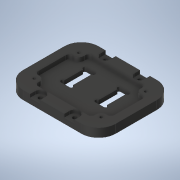
# Autodesk Inventor part: カメラ_メインフレーム1_KCSU5380
Saved by Autodesk Inventor 2020.3 (Build 243373000, 373)
## iProperties
Created: 2018-06-08
Part Number: カメラ_メインフレーム1_KCSU5380
Material: アセタール樹脂、黒
Document SubType Name: Modeling
Designer: taka
Density: 1.425 g/cm^3
Appearance: 滑らか - 黒
Mass: 10.5319 g
Surface Area: 59.4191 cm^2
Volume: 7.39082 cm^3
Category: 頭
Author: taka
Autodesk Inventor part; units mm, degrees
ref_plane "YZ Plane" through (0, 0, 0) normal (1, 0, 0) x (0, 1, 0)
ref_plane "XZ Plane" through (0, 0, 0) normal (0, 1, 0) x (-1, 0, 0)
ref_plane "XY Plane" through (0, 0, 0) normal (0, 0, 1) x (1, 0, 0)
derived "カメラ_メインフレーム1_基礎.ipt"
sketch "スケッチ1" plane through (0, 0, 0) normal (0, 1, 0) x (-1, 0, 0)
  line L0 (0, 0) -> (44, 0)
  line L1 (44, 0) -> (44, -54)
  line L2 (44, -54) -> (0, -54)
  line L3 (0, -54) -> (0, 0)
  line L4 (32.5, -14.5) -> (17.5, -14.5) construction
  line L5 (17.5, -14.5) -> (17.5, -19.5) construction
  line L6 (17.5, -19.5) -> (32.5, -19.5) construction
  line L7 (32.5, -19.5) -> (32.5, -14.5) construction
  line L8 (32.5, -34.5) -> (17.5, -34.5) construction
  line L9 (17.5, -34.5) -> (17.5, -39.5) construction
  line L10 (17.5, -39.5) -> (32.5, -39.5) construction
  line L11 (32.5, -39.5) -> (32.5, -34.5) construction
  line L12 (32.55, -19.55) -> (17.45, -19.55)
  line L13 (17.45, -19.55) -> (17.45, -14.45)
  line L14 (17.45, -14.45) -> (32.55, -14.45)
  line L15 (32.55, -14.45) -> (32.55, -19.55)
  line L16 (17.45, -34.45) -> (32.55, -34.45)
  line L17 (32.55, -34.45) -> (32.55, -39.55)
  line L18 (32.55, -39.55) -> (17.45, -39.55)
  line L19 (17.45, -39.55) -> (17.45, -34.45)
  circle A0 centre (31.5, -19.55) radius 1.05
  circle A1 centre (31.5, -14.45) radius 1.05
  circle A2 centre (18.5, -19.55) radius 1.05
  circle A3 centre (18.5, -14.45) radius 1.05
  circle A4 centre (18.5, -34.45) radius 1.05
  circle A5 centre (18.5, -39.55) radius 1.05
  circle A6 centre (31.5, -34.45) radius 1.05
  circle A7 centre (31.5, -39.55) radius 1.05
  circle A8 centre (35, -7.5) radius 0.8
  circle A9 centre (35, -46.5) radius 0.8
  circle A10 centre (9, -7.5) radius 0.8
  circle A11 centre (9, -46.5) radius 0.8
  circle A12 centre (41, -17) radius 1.15
  circle A13 centre (41, -37) radius 1.15
  line L20 (44, -14.5) -> (0, -14.5) construction
  line L21 (0, -14.5) -> (0, -19.5) construction
  line L22 (0, -19.5) -> (44, -19.5) construction
  line L23 (44, -19.5) -> (44, -14.5)
  circle A14 centre (3, -17) radius 1.15
  circle A15 centre (3, -37) radius 1.15
  line L24 (44, -34.5) -> (0, -34.5) construction
  line L25 (0, -34.5) -> (0, -39.5) construction
  line L26 (0, -39.5) -> (44, -39.5) construction
  line L27 (44, -39.5) -> (44, -34.5)
  line L28 (38, -4.5) -> (6, -4.5) construction
  line L29 (6, -4.5) -> (6, -49.5) construction
  line L30 (6, -49.5) -> (38, -49.5) construction
  line L31 (38, -49.5) -> (38, -4.5) construction
  circle A16 centre (22, -27) radius 7.5 construction
  line L32 (29.5, -13) -> (14.5, -13) construction
  line L33 (14.5, -13) -> (14.5, -53) construction
  line L34 (14.5, -53) -> (29.5, -53) construction
  line L35 (29.5, -53) -> (29.5, -13) construction
  circle A17 centre (22, -27) radius 6.5 construction
  circle A18 centre (26.5, -50) radius 0.9
  circle A19 centre (17.5, -16) radius 0.9
extrude "押し出し1" add sketch "スケッチ1" along normal blind 5 contours L0 L1 L2 L3 | A19 L13 | A18
fillet "フィレット1" radius 10 4 edges at (0, 2.5, -54) (0, 2.5, 0) (-44, 2.5, -54) (-44, 2.5, 0)
sketch "スケッチ4" plane through (-34, 5, 0) normal (0, 1, 0) x (1, 0, 0)
  circle A0 centre (-1, 7.5) radius 3
  circle A1 centre (-1, 46.5) radius 3
  circle A2 centre (25, 46.5) radius 3
  circle A3 centre (25, 7.5) radius 3
  circle A4 centre (-1, 7.5) radius 0.8 projected
  circle A5 centre (-1, 46.5) radius 0.8 projected
  circle A6 centre (25, 46.5) radius 0.8 projected
  circle A7 centre (25, 7.5) radius 0.8 projected
  line L0 (-3.7272, 8.75) -> (-3.7272, 45.25)
  line L1 (27.7272, 8.75) -> (27.7272, 45.25)
  line L2 (0.25, 49.2272) -> (23.75, 49.2272)
  line L3 (0.25, 4.7728) -> (23.75, 4.7728)
  point P0 (34, 0)
  dimension "d16" = 6
  dimension "d17" = 6
  dimension "d18" = 6
  dimension "d19" = 6
  constraints: 8 end point, 8 point on circle, 4 centre point, 4 concentric, 2 parallel, 1 perpendicular, 1 vertical
  measures "d16" diameter of A0
  measures "d17" diameter of A1
  measures "d18" diameter of A2
  measures "d19" diameter of A3
extrude "押し出し4" cut sketch "スケッチ4" against normal blind 2.6 contours A0 L0 A1 L2 A2 L1 A3 L3
sketch "スケッチ5" plane through (-34, 5, 0) normal (0, 1, 0) x (1, 0, 0)
  circle A0 centre (-7, 17) radius 3
  circle A1 centre (-7, 37) radius 3
  circle A2 centre (31, 17) radius 3
  circle A3 centre (31, 37) radius 3
  circle A4 centre (-7, 17) radius 1.15 projected
  circle A5 centre (-7, 37) radius 1.15 projected
  circle A6 centre (31, 37) radius 1.15 projected
  circle A7 centre (31, 17) radius 1.15 projected
  line L0 (-7, 20) -> (-10, 20)
  line L1 (-7, 14) -> (-10, 14)
  line L2 (31, 14) -> (34, 14)
  line L3 (31, 20) -> (34, 20)
  line L4 (31, 34) -> (34, 34)
  line L5 (31, 40) -> (34, 40)
  line L6 (-10, 14) -> (-10, 20)
  line L7 (34, 14) -> (34, 20)
  line L8 (34, 34) -> (34, 40)
  line L9 (-7, 34) -> (-10, 34)
  line L10 (-10, 34) -> (-10, 40)
  line L11 (-10, 40) -> (-7, 40)
  point P0 (34, 0)
  dimension "d22" = 6
  dimension "d23" = 6
  dimension "d24" = 6
  dimension "d25" = 6
  constraints: 24 end point, 8 point on circle, 7 horizontal, 7 tangent, 4 centre point, 4 concentric, 2 perpendicular, 1 collinear, 1 vertical
  measures "d22" diameter of A0
  measures "d23" diameter of A1
  measures "d24" diameter of A2
  measures "d25" diameter of A3
extrude "押し出し5" cut sketch "スケッチ5" against normal blind 2
fillet "フィレット2" radius 2 8 edges at (-33.75, 3.7, -4.7728) (-37.7272, 3.7, -8.75) (-6.2728, 3.7, -8.75) (-10.25, 3.7, -4.7728) (-6.2728, 3.7, -45.25) (-10.25, 3.7, -49.2272) (-33.75, 3.7, -49.2272) (-37.7272, 3.7, -45.25)
